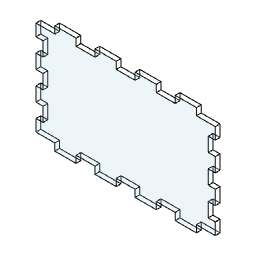
case_5_3mm (Autodesk Fusion 360 design; units mm, degrees)
Autodesk Fusion 360 part; units mm, degrees
sketch "スケッチ1" plane through (0, 0, 0) normal (0, 1, 0) x (1, 0, 0)
  line L0 (0, 0) -> (74, 0)
  line L1 (74, 0) -> (74, -44)
  line L2 (74, -44) -> (0, -44)
  line L3 (0, -44) -> (0, 0)
  dimension "d1" = 74
  dimension "d2" = 44
  constraint horizontal L0
  constraint vertical L1
  constraint horizontal L2
  constraint vertical L3
  constraint coincident L0.start L3.end
  measures "d1" distance of L0.start L0.end
  measures "d2" distance of L0.start L2.end
extrude "押し出し1" add sketch "スケッチ1" along normal blind 2
sketch "スケッチ2" plane through (0, 0, 0) normal (0, -1, 0) x (1, 0, 0)
  line L0 (74, 44) -> (0, 44)
  line L1 (0, 44) -> (0, 0)
  line L2 (0, 0) -> (74, 0)
  line L3 (74, 0) -> (74, 44)
  line L4 (72, 37) -> (74, 37)
  line L5 (74, 37) -> (74, 31)
  line L6 (74, 31) -> (72, 31)
  line L7 (72, 31) -> (72, 37)
  line L8 (74, 25) -> (74, 19)
  line L9 (74, 19) -> (72, 19)
  line L10 (72, 19) -> (72, 25)
  line L11 (72, 25) -> (74, 25)
  line L12 (74, 13) -> (74, 7)
  line L13 (74, 7) -> (72, 7)
  line L14 (72, 7) -> (72, 13)
  line L15 (72, 13) -> (74, 13)
  line L16 (2, 25) -> (2, 19)
  line L17 (2, 31) -> (0, 31)
  line L18 (2, 37) -> (2, 31)
  line L19 (0, 25) -> (2, 25)
  line L20 (2, 13) -> (2, 7)
  line L21 (0, 19) -> (0, 25)
  line L22 (0, 13) -> (2, 13)
  line L23 (2, 7) -> (0, 7)
  line L24 (0, 31) -> (0, 37)
  line L25 (0, 37) -> (2, 37)
  line L26 (0, 7) -> (0, 13)
  line L27 (2, 19) -> (0, 19)
  line L28 (74, 44) -> (72, 44)
  line L29 (72, 44) -> (72, 42)
  line L30 (72, 42) -> (74, 42)
  line L31 (74, 42) -> (74, 44)
  line L32 (0, 44) -> (2, 44)
  line L33 (2, 44) -> (2, 42)
  line L34 (2, 42) -> (0, 42)
  line L35 (0, 42) -> (0, 44)
  line L36 (0, 0) -> (2, 0)
  line L37 (2, 0) -> (2, 2)
  line L38 (2, 2) -> (0, 2)
  line L39 (0, 2) -> (0, 0)
  line L40 (74, 0) -> (72, 0)
  line L41 (72, 0) -> (72, 2)
  line L42 (72, 2) -> (74, 2)
  line L43 (74, 2) -> (74, 0)
  dimension "d7" = 0
  dimension "d8" = -12
  dimension "d9" = 2
  dimension "d10" = 7
  dimension "d11" = 6
  dimension "d12" = 6
  dimension "d13" = 7
  dimension "d16" = -72
  dimension "d17" = 0
  constraint horizontal L4
  constraint vertical L5
  constraint horizontal L6
  constraint vertical L7
  constraint coincident L3 L5.end
  constraint horizontal L28
  constraint vertical L29
  constraint horizontal L30
  constraint vertical L31
  constraint coincident L0.start L3.end
  constraint horizontal L32
  constraint vertical L33
  constraint horizontal L34
  constraint vertical L35
  constraint coincident L0.end L1.start
  constraint horizontal L36
  constraint vertical L37
  constraint horizontal L38
  constraint vertical L39
  constraint coincident L1.end L2.start
  constraint horizontal L40
  constraint vertical L41
  constraint horizontal L42
  constraint vertical L43
  constraint coincident L2.end L3.start
  measures "d9" distance of L4.start L4.end
  measures "d10" distance of L0 L4
  measures "d11" distance of L4.end L5.end
  measures "d12" distance of L6 L11
  measures "d13" distance of L2 L13
extrude "押し出し2" cut sketch "スケッチ2" against normal blind 2 contours L0 L3 L28 L29 L30 L31 | L0 L1 L32 L33 L34 L35 | L3 L4 L5 L6 L7 | L3 L8 L9 L10 L11 | L1 L17 L18 L24 L25 | L3 L12 L13 L14 L15 | L1 L16 L19 L21 L27 | L2 L3 L40 L41 L42 L43 | L1 L20 L22 L23 L26 | L1 L2 L36 L37 L38 L39
sketch "スケッチ3" plane through (0, 0, 0) normal (0, -1, 0) x (1, 0, 0)
  line L0 (74, 31) -> (72, 31)
  line L1 (72, 31) -> (72, 37)
  line L2 (72, 37) -> (74, 37)
  line L3 (74, 37) -> (74, 42)
  line L4 (74, 42) -> (72, 42)
  line L5 (72, 42) -> (72, 44)
  line L6 (72, 44) -> (2, 44)
  line L7 (2, 44) -> (2, 42)
  line L8 (2, 42) -> (0, 42)
  line L9 (0, 42) -> (0, 37)
  line L10 (0, 37) -> (2, 37)
  line L11 (2, 37) -> (2, 31)
  line L12 (2, 31) -> (0, 31)
  line L13 (0, 31) -> (0, 25)
  line L14 (0, 25) -> (2, 25)
  line L15 (2, 25) -> (2, 19)
  line L16 (2, 19) -> (0, 19)
  line L17 (0, 19) -> (0, 13)
  line L18 (0, 13) -> (2, 13)
  line L19 (2, 13) -> (2, 7)
  line L20 (2, 7) -> (0, 7)
  line L21 (0, 7) -> (0, 2)
  line L22 (0, 2) -> (2, 2)
  line L23 (2, 2) -> (2, 0)
  line L24 (2, 0) -> (72, 0)
  line L25 (72, 0) -> (72, 2)
  line L26 (72, 2) -> (74, 2)
  line L27 (74, 2) -> (74, 7)
  line L28 (74, 7) -> (72, 7)
  line L29 (72, 7) -> (72, 13)
  line L30 (72, 13) -> (74, 13)
  line L31 (74, 13) -> (74, 19)
  line L32 (74, 19) -> (72, 19)
  line L33 (72, 19) -> (72, 25)
  line L34 (72, 25) -> (74, 25)
  line L35 (74, 25) -> (74, 31)
  line L36 (0, 44) -> (7, 44)
  line L37 (7, 44) -> (7, 42)
  line L38 (7, 42) -> (0, 42)
  line L39 (0, 42) -> (0, 44)
  line L40 (16, 42) -> (24, 42)
  line L41 (24, 42) -> (24, 44)
  line L42 (24, 44) -> (16, 44)
  line L43 (16, 44) -> (16, 42)
  line L44 (41, 42) -> (41, 44)
  line L45 (33, 42) -> (41, 42)
  line L46 (41, 44) -> (33, 44)
  line L47 (33, 44) -> (33, 42)
  line L48 (58, 42) -> (58, 44)
  line L49 (50, 42) -> (58, 42)
  line L50 (58, 44) -> (50, 44)
  line L51 (50, 44) -> (50, 42)
  line L52 (67, 42) -> (74, 42)
  line L53 (74, 42) -> (74, 44)
  line L54 (74, 44) -> (67, 44)
  line L55 (67, 44) -> (67, 42)
  line L56 (7, 0) -> (0, 0)
  line L57 (41, 2) -> (33, 2)
  line L58 (33, 2) -> (33, 0)
  line L59 (50, 2) -> (50, 0)
  line L60 (24, 2) -> (16, 2)
  line L61 (24, 0) -> (24, 2)
  line L62 (16, 0) -> (24, 0)
  line L63 (7, 2) -> (7, 0)
  line L64 (50, 0) -> (58, 0)
  line L65 (67, 2) -> (67, 0)
  line L66 (0, 0) -> (0, 2)
  line L67 (74, 2) -> (67, 2)
  line L68 (41, 0) -> (41, 2)
  line L69 (58, 2) -> (50, 2)
  line L70 (16, 2) -> (16, 0)
  line L71 (33, 0) -> (41, 0)
  line L72 (67, 0) -> (74, 0)
  line L73 (58, 0) -> (58, 2)
  line L74 (0, 2) -> (7, 2)
  line L75 (74, 0) -> (74, 2)
  line L76 (72, 0) -> (72, 2)
  line L77 (74, 0) -> (72, 0)
  line L78 (2, 2) -> (2, 0)
  line L79 (2, 0) -> (0, 0)
  dimension "d20" = 8
  dimension "d21" = 2
  dimension "d22" = 2
  dimension "d23" = 9
  dimension "d26" = 17
  dimension "d27" = 0
  dimension "d28" = 2
  dimension "d29" = 9
  constraint horizontal L36
  constraint vertical L37
  constraint horizontal L38
  constraint vertical L39
  constraint horizontal L40
  constraint vertical L41
  constraint horizontal L42
  constraint vertical L43
  constraint coincident L6 L41.end
  constraint horizontal L52
  constraint vertical L53
  constraint horizontal L54
  constraint vertical L55
  measures "d20" distance of L40.start L40.end
  measures "d21" distance of L40.start L42.end
  measures "d22" distance of L36.start L8.end
  measures "d23" distance of L37 L43
  measures "d28" distance of L3.end L53.end
  measures "d29" distance of L48 L55
extrude "押し出し3" cut sketch "スケッチ3" against normal blind 2 contours L4 L5 L52 L53 L54 | L5 L6 L52 L54 L55 | L6 L48 L49 L50 L51 | L25 L26 L67 L72 L75 L76 L77 | L6 L44 L45 L46 L47 | L24 L25 L65 L67 L72 L76 | L6 L40 L41 L42 L43 | L24 L59 L64 L69 L73 | L6 L7 L36 L37 L38 | L7 L8 L36 L38 L39 | L24 L57 L58 L68 L71 | L24 L60 L61 L62 L70 | L23 L24 L56 L63 L74 L78 | L22 L23 L56 L66 L74 L78 L79
sketch "スケッチ4" plane through (0, 0, 0) normal (0, -1, 0) x (1, 0, 0)
  line L0 (41, 2) -> (41, 0)
  line L1 (41, 0) -> (50, 0)
  line L2 (50, 0) -> (50, 2)
  line L3 (50, 2) -> (58, 2)
  line L4 (58, 2) -> (58, 0)
  line L5 (58, 0) -> (67, 0)
  line L6 (67, 0) -> (67, 2)
  line L7 (67, 2) -> (74, 2)
  line L8 (74, 2) -> (74, 7)
  line L9 (74, 7) -> (72, 7)
  line L10 (72, 7) -> (72, 13)
  line L11 (72, 13) -> (74, 13)
  line L12 (74, 13) -> (74, 19)
  line L13 (74, 19) -> (72, 19)
  line L14 (72, 19) -> (72, 25)
  line L15 (72, 25) -> (74, 25)
  line L16 (74, 25) -> (74, 31)
  line L17 (74, 31) -> (72, 31)
  line L18 (72, 31) -> (72, 37)
  line L19 (72, 37) -> (74, 37)
  line L20 (74, 37) -> (74, 42)
  line L21 (74, 42) -> (67, 42)
  line L22 (67, 42) -> (67, 44)
  line L23 (67, 44) -> (58, 44)
  line L24 (58, 44) -> (58, 42)
  line L25 (58, 42) -> (50, 42)
  line L26 (50, 42) -> (50, 44)
  line L27 (50, 44) -> (41, 44)
  line L28 (41, 44) -> (41, 42)
  line L29 (41, 42) -> (33, 42)
  line L30 (33, 42) -> (33, 44)
  line L31 (33, 44) -> (24, 44)
  line L32 (24, 44) -> (24, 42)
  line L33 (24, 42) -> (16, 42)
  line L34 (16, 42) -> (16, 44)
  line L35 (16, 44) -> (7, 44)
  line L36 (7, 44) -> (7, 42)
  line L37 (7, 42) -> (0, 42)
  line L38 (0, 42) -> (0, 37)
  line L39 (0, 37) -> (2, 37)
  line L40 (2, 37) -> (2, 31)
  line L41 (2, 31) -> (0, 31)
  line L42 (0, 31) -> (0, 25)
  line L43 (0, 25) -> (2, 25)
  line L44 (2, 25) -> (2, 19)
  line L45 (2, 19) -> (0, 19)
  line L46 (0, 19) -> (0, 13)
  line L47 (0, 13) -> (2, 13)
  line L48 (2, 13) -> (2, 7)
  line L49 (2, 7) -> (0, 7)
  line L50 (0, 7) -> (0, 2)
  line L51 (0, 2) -> (7, 2)
  line L52 (7, 2) -> (7, 0)
  line L53 (7, 0) -> (16, 0)
  line L54 (16, 0) -> (16, 2)
  line L55 (16, 2) -> (24, 2)
  line L56 (24, 2) -> (24, 0)
  line L57 (24, 0) -> (33, 0)
  line L58 (33, 0) -> (33, 2)
  line L59 (33, 2) -> (41, 2)
  line L60 (7, 45) -> (16, 45)
  line L61 (16, 45) -> (16, 44)
  line L62 (16, 44) -> (7, 44)
  line L63 (7, 44) -> (7, 45)
  line L64 (24, 45) -> (33, 45)
  line L65 (33, 45) -> (33, 44)
  line L66 (33, 44) -> (24, 44)
  line L67 (24, 44) -> (24, 45)
  line L68 (41, 45) -> (50, 45)
  line L69 (50, 45) -> (50, 44)
  line L70 (50, 44) -> (41, 44)
  line L71 (41, 44) -> (41, 45)
  line L72 (58, 45) -> (67, 45)
  line L73 (67, 45) -> (67, 44)
  line L74 (67, 44) -> (58, 44)
  line L75 (58, 44) -> (58, 45)
  line L76 (74, 42) -> (75, 42)
  line L77 (75, 42) -> (75, 37)
  line L78 (75, 37) -> (74, 37)
  line L79 (74, 37) -> (74, 42)
  line L80 (74, 31) -> (75, 31)
  line L81 (75, 31) -> (75, 25)
  line L82 (75, 25) -> (74, 25)
  line L83 (74, 25) -> (74, 31)
  line L84 (74, 19) -> (75, 19)
  line L85 (75, 19) -> (75, 13)
  line L86 (75, 13) -> (74, 13)
  line L87 (74, 13) -> (74, 19)
  line L88 (74, 7) -> (75, 7)
  line L89 (75, 7) -> (75, 2)
  line L90 (75, 2) -> (74, 2)
  line L91 (74, 2) -> (74, 7)
  line L92 (58, -1) -> (67, -1)
  line L93 (67, -1) -> (67, 0)
  line L94 (67, 0) -> (58, 0)
  line L95 (58, 0) -> (58, -1)
  line L96 (41, -1) -> (50, -1)
  line L97 (50, -1) -> (50, 0)
  line L98 (50, 0) -> (41, 0)
  line L99 (41, 0) -> (41, -1)
  line L100 (24, 0) -> (33, 0)
  line L101 (33, 0) -> (33, -1)
  line L102 (33, -1) -> (24, -1)
  line L103 (24, -1) -> (24, 0)
  line L104 (16, -1) -> (7, -1)
  line L105 (7, -1) -> (7, 0)
  line L106 (7, 0) -> (16, 0)
  line L107 (16, 0) -> (16, -1)
  line L108 (0, 2) -> (-1, 2)
  line L109 (-1, 2) -> (-1, 7)
  line L110 (-1, 7) -> (0, 7)
  line L111 (0, 7) -> (0, 2)
  line L112 (0, 13) -> (-1, 13)
  line L113 (-1, 13) -> (-1, 19)
  line L114 (-1, 19) -> (0, 19)
  line L115 (0, 19) -> (0, 13)
  line L116 (0, 25) -> (-1, 25)
  line L117 (-1, 25) -> (-1, 31)
  line L118 (-1, 31) -> (0, 31)
  line L119 (0, 31) -> (0, 25)
  line L120 (0, 37) -> (-1, 37)
  line L121 (-1, 37) -> (-1, 42)
  line L122 (-1, 42) -> (0, 42)
  line L123 (0, 42) -> (0, 37)
  constraint horizontal L60
  constraint vertical L61
  constraint horizontal L62
  constraint vertical L63
  constraint coincident L34.end L35.start
  constraint horizontal L64
  constraint vertical L65
  constraint horizontal L66
  constraint vertical L67
  constraint coincident L30.end L31.start
  constraint horizontal L68
  constraint vertical L69
  constraint horizontal L70
  constraint vertical L71
  constraint coincident L26.end L27.start
  constraint horizontal L72
  constraint vertical L73
  constraint horizontal L74
  constraint vertical L75
  constraint coincident L22.end L23.start
  constraint horizontal L76
  constraint vertical L77
  constraint horizontal L78
  constraint vertical L79
  constraint coincident L20.end L21.start
  constraint horizontal L80
  constraint vertical L81
  constraint horizontal L82
  constraint vertical L83
  constraint coincident L16.end L17.start
  constraint horizontal L84
  constraint vertical L85
  constraint horizontal L86
  constraint vertical L87
  constraint coincident L12.end L13.start
  constraint horizontal L88
  constraint vertical L89
  constraint horizontal L90
  constraint vertical L91
  constraint coincident L8.end L9.start
  constraint horizontal L92
  constraint vertical L93
  constraint horizontal L94
  constraint vertical L95
  constraint coincident L5.end L6.start
  constraint horizontal L96
  constraint vertical L97
  constraint horizontal L98
  constraint vertical L99
  constraint coincident L1.end L2.start
  constraint horizontal L100
  constraint vertical L101
  constraint horizontal L102
  constraint vertical L103
  constraint coincident L56.end L57.start
  constraint horizontal L104
  constraint vertical L105
  constraint horizontal L106
  constraint vertical L107
  constraint coincident L52.end L53.start
  constraint horizontal L108
  constraint vertical L109
  constraint horizontal L110
  constraint vertical L111
  constraint coincident L50.end L51.start
  constraint horizontal L112
  constraint vertical L113
  constraint horizontal L114
  constraint vertical L115
  constraint coincident L46.end L47.start
  constraint horizontal L116
  constraint vertical L117
  constraint horizontal L118
  constraint vertical L119
  constraint coincident L42.end L43.start
  constraint horizontal L120
  constraint vertical L121
  constraint horizontal L122
  constraint vertical L123
  constraint coincident L38.end L39.start
extrude "押し出し4" add sketch "スケッチ4" against normal blind 2 contours L1 L96 L97 L98 L99 | L57 L100 L101 L102 L103 | L5 L92 L93 L94 L95 | L53 L104 L105 L106 L107 | L8 L88 L89 L90 L91 | L50 L108 L109 L110 L111 | L12 L84 L85 L86 L87 | L46 L112 L113 L114 L115 | L16 L80 L81 L82 L83 | L42 L116 L117 L118 L119 | L20 L76 L77 L78 L79 | L38 L120 L121 L122 L123 | L23 L72 L73 L74 L75 | L35 L60 L61 L62 L63 | L27 L68 L69 L70 L71 | L31 L64 L65 L66 L67
sketch "スケッチ5" plane through (0, 0, 0) normal (0, -1, 0) x (1, 0, 0)
  line L0 (41, 2) -> (41, -1)
  line L1 (41, -1) -> (50, -1)
  line L2 (50, -1) -> (50, 2)
  line L3 (50, 2) -> (58, 2)
  line L4 (58, 2) -> (58, -1)
  line L5 (58, -1) -> (67, -1)
  line L6 (67, -1) -> (67, 2)
  line L7 (67, 2) -> (75, 2)
  line L8 (75, 2) -> (75, 7)
  line L9 (75, 7) -> (72, 7)
  line L10 (72, 7) -> (72, 13)
  line L11 (72, 13) -> (75, 13)
  line L12 (75, 13) -> (75, 19)
  line L13 (75, 19) -> (72, 19)
  line L14 (72, 19) -> (72, 25)
  line L15 (72, 25) -> (75, 25)
  line L16 (75, 25) -> (75, 31)
  line L17 (75, 31) -> (72, 31)
  line L18 (72, 31) -> (72, 37)
  line L19 (72, 37) -> (75, 37)
  line L20 (75, 37) -> (75, 42)
  line L21 (75, 42) -> (67, 42)
  line L22 (67, 42) -> (67, 45)
  line L23 (67, 45) -> (58, 45)
  line L24 (58, 45) -> (58, 42)
  line L25 (58, 42) -> (50, 42)
  line L26 (50, 42) -> (50, 45)
  line L27 (50, 45) -> (41, 45)
  line L28 (41, 45) -> (41, 42)
  line L29 (41, 42) -> (33, 42)
  line L30 (33, 42) -> (33, 45)
  line L31 (33, 45) -> (24, 45)
  line L32 (24, 45) -> (24, 42)
  line L33 (24, 42) -> (16, 42)
  line L34 (16, 42) -> (16, 45)
  line L35 (16, 45) -> (7, 45)
  line L36 (7, 45) -> (7, 42)
  line L37 (7, 42) -> (-1, 42)
  line L38 (-1, 42) -> (-1, 37)
  line L39 (-1, 37) -> (2, 37)
  line L40 (2, 37) -> (2, 31)
  line L41 (2, 31) -> (-1, 31)
  line L42 (-1, 31) -> (-1, 25)
  line L43 (-1, 25) -> (2, 25)
  line L44 (2, 25) -> (2, 19)
  line L45 (2, 19) -> (-1, 19)
  line L46 (-1, 19) -> (-1, 13)
  line L47 (-1, 13) -> (2, 13)
  line L48 (2, 13) -> (2, 7)
  line L49 (2, 7) -> (-1, 7)
  line L50 (-1, 7) -> (-1, 2)
  line L51 (-1, 2) -> (7, 2)
  line L52 (7, 2) -> (7, -1)
  line L53 (7, -1) -> (16, -1)
  line L54 (16, -1) -> (16, 2)
  line L55 (16, 2) -> (24, 2)
  line L56 (24, 2) -> (24, -1)
  line L57 (24, -1) -> (33, -1)
  line L58 (33, -1) -> (33, 2)
  line L59 (33, 2) -> (41, 2)
